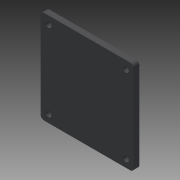
# Autodesk Inventor part: Batt_Plate_FPV
Saved by Autodesk Inventor 2015 (Build 190159000, 159)
## iProperties
Created: 2017-02-15
Part Number: Batt_Plate_FPV
Material: Generic
Document SubType Name: Modeling
Designer: Hampus
Density: 1 g/cm^3
Appearance: Gray
Author: Hampus
Autodesk Inventor part; units mm, degrees
ref_plane "YZ Plane" through (0, 0, 0) normal (1, 0, 0) x (0, 1, 0)
ref_plane "XZ Plane" through (0, 0, 0) normal (0, 1, 0) x (-1, 0, 0)
ref_plane "XY Plane" through (0, 0, 0) normal (0, 0, 1) x (1, 0, 0)
sketch "Sketch3" plane through (0, 0, 0) normal (0, 1, 0) x (-1, 0, 0)
  line L0 (-15, 0) -> (-2, 0)
  line L1 (0, -2) -> (0, -48)
  line L2 (-2, -50) -> (-48, -50)
  line L3 (-50, -48) -> (-50, -2)
  circle A0 centre (-4.2426, -4.2426) radius 1.5
  circle A1 centre (-4.2426, -45.7574) radius 1.5
  circle A2 centre (-45.7574, -45.7574) radius 1.5
  circle A3 centre (-45.7574, -4.2426) radius 1.5
  line L4 (-35, 0) -> (-48, 0)
  arc A4 (0, -2) -> (-2, 0) centre (-2, -2) ccw
  arc A5 (-48, 0) -> (-50, -2) centre (-48, -2) ccw
  arc A6 (-50, -48) -> (-48, -50) centre (-48, -48) ccw
  arc A7 (-2, -50) -> (0, -48) centre (-2, -48) ccw
  line L5 (-48, 0) -> (-2, 0)
  point P0 (0, 0)
  point P1 (0, 0)
  point P2 (-50, 0)
  point P3 (0, 0)
  point P4 (0, -50)
  dimension "d19" = 50
  dimension "d20" = 50
  dimension "d21" = 3
  dimension "d22" = 3
  dimension "d23" = 3
  dimension "d24" = 3
  dimension "d32" = 2
  constraints: 12 end point, 8 centre point, 8 point on circle, 8 tangent, 7 point on line, 2 parallel, 2 perpendicular, 1 collinear
  measures "d19" distance of point (0, 0) point (0, -50)
  measures "d20" distance of point (-50, 0) point (0, 0)
  measures "d21" diameter of A0
  measures "d22" diameter of A1
  measures "d23" diameter of A2
  measures "d24" diameter of A3
  measures "d32" radius of A4
extrude "Extrusion2" add sketch "Sketch3" along normal blind 3
body "Solid2"
